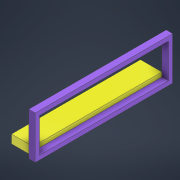
# Autodesk Inventor part: 110033226_ipt_20_塔樓窗戶
Saved by Autodesk Inventor 2022 (Build 260153000, 153)
## iProperties
Created: 2022-06-23
Part Number: 110033226_ipt_20_塔樓窗戶
Material: 一般
Document SubType Name: Modeling
Designer: User
Density: 1 g/cm^3
Appearance: 預設
Author: User
Autodesk Inventor part; units mm, degrees
ref_plane "YZ Plane" through (0, 0, 0) normal (1, 0, 0) x (0, 1, 0)
ref_plane "XZ Plane" through (0, 0, 0) normal (0, 1, 0) x (-1, 0, 0)
ref_plane "XY Plane" through (0, 0, 0) normal (0, 0, 1) x (1, 0, 0)
sketch "草圖1" plane through (0, 0, 0) normal (0, 1, 0) x (-1, 0, 0)
  line L0 (2.5, 15) -> (-2.5, 15)
  line L1 (-2.5, 15) -> (-2.5, -15)
  line L2 (-2.5, -15) -> (2.5, -15)
  line L3 (2.5, -15) -> (2.5, 15)
  circle A0 centre (0, 12.5) radius 1.7
  circle A1 centre (0, 7.5) radius 1.7
  circle A2 centre (0, 2.5) radius 1.7
  circle A3 centre (0, -2.5) radius 1.7
  circle A4 centre (0, -7.5) radius 1.7
  circle A5 centre (0, -12.5) radius 1.7
  point P0 (0, 0)
  point P1 (2.5, 0)
  point P2 (0, 15)
  dimension "d0" = 5
  dimension "d1" = 30
  dimension "d2" = 3.4
  dimension "d3" = 2.5
  dimension "d4" = 2.5
  dimension "d7" = 5
  constraints: 8 end point, 6 centre point, 2 midpoint, 2 parallel, 1 horizontal, 1 horizontal alignment, 1 perpendicular, 1 vertical, 1 vertical alignment, 10 other
  measures "d0" distance of L2.end L1.end
  measures "d1" distance of L1.end L0.end
  measures "d2" diameter of A0
  measures "d3" distance from line of L3 A0.centre
  measures "d4" distance from line of L0 A0.centre
  measures "d7" distance of A0.centre A1.centre
extrude "擠出1" add sketch "草圖1" along normal blind 2 contours L3 L2 L1 L0 | A0 | A1 | A2 | A3 | A4 | A5
extrude "擠出2" cut sketch "草圖1" along normal blind 1.5 contours A0 | A1 | A2 | A3 | A4 | A5
sketch "草圖2" plane through (2.5, 0, 15) normal (1, 0, 0) x (0, 0, -1)
  line L0 (-1, 10) -> (31, 10)
  line L1 (31, 10) -> (31, 0)
  line L2 (31, 0) -> (-1, 0)
  line L3 (-1, 0) -> (-1, 10)
  line L4 (0, 0) -> (30, 0) projected
  line L5 (30, 9) -> (0, 9)
  line L6 (0, 9) -> (0, 1)
  line L7 (0, 1) -> (30, 1)
  line L8 (30, 1) -> (30, 9)
  point P0 (15, 0)
  point P1 (15, 10)
  point P2 (15, 0)
  point P3 (15, 0)
  dimension "d16" = 32
  dimension "d17" = 10
  dimension "d18" = 1
  constraints: 16 end point, 4 midpoint, 4 parallel, 2 perpendicular, 1 horizontal, 1 vertical alignment, 3 other
  measures "d16" distance of L1.end L2.end
  measures "d17" distance of L0.end L1.end
  measures "d18" distance between parallel lines of L0 L5
extrude "擠出3" add sketch "草圖2" along normal blind 1.5
